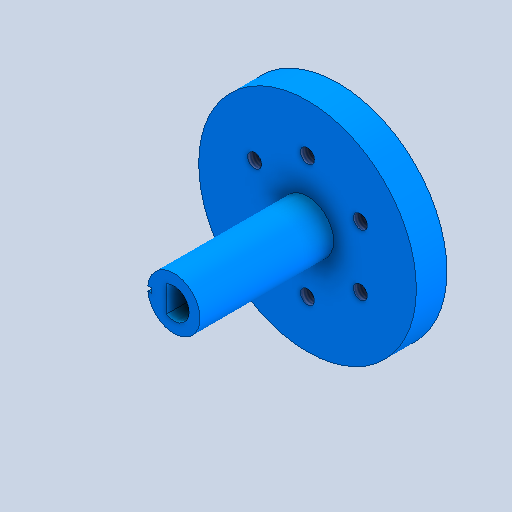
# Autodesk Inventor part: E_01
Saved by Autodesk Inventor 2024.3 (Build 283343000, 343)
## iProperties
Created: 2021-11-18
Part Number: E_01
Material: PETG
Document SubType Name: Modeling
Designer: Alcatraz
Density: 1.27 g/cm^3
Appearance: Genérico
Author: Alcatraz
Autodesk Inventor part; units mm, degrees
sketch "Boceto1" plane through (0, 0, 0) normal (0, 0, 1) x (1, 0, 0)
  circle A0 centre (0, 0) radius 28.5
  dimension "DiametroJunta" = 57
  constraints: 1 centre point, 1 coincident
  measures "DiametroJunta" diameter of A0
extrude "Extrusión1" add sketch "Boceto1" along normal blind 8
sketch "Boceto2" plane through (0, 0, 8) normal (0, 0, 1) x (1, 0, 0)
  circle A0 centre (0, 0) radius 6.8425
  dimension "DiametroEje" = 13.685
  constraints: 1 centre point, 1 coincident
  measures "DiametroEje" diameter of A0
extrude "Extrusión2" add sketch "Boceto2" along normal blind 35
sketch "Boceto3" plane through (0, 0, 43) normal (0, 0, 1) x (1, 0, 0)
  arc A0 (-2, -3.4641) -> (-2, 3.4641) centre (0, 0) ccw
  line L0 (-2, 3.4641) -> (-2, -3.4641)
  circle A1 centre (0, 0) radius 6.8425 projected
  point P0 (2, -3.4641)
  point P1 (2, 3.4641)
  dimension "DiametroEntrada" = 8
  dimension "d21" = 2
  constraints: 4 point on circle, 2 end point, 1 centre point, 1 coincident, 1 concentric, 1 vertical
  measures "DiametroEntrada" diameter of A0
  measures "d21" distance from line of point (0, 0) L0
extrude "Extrusión3" cut sketch "Boceto3" against normal blind 34.5 contours L0 A0
ref_plane "Plano de trabajo1" through (6.8425, 0, 8) normal (1, 0, 0) x (0, 1, 0)
ref_plane "Plano de trabajo2" through (-6.8425, 0, 8) normal (1, 0, 0) x (0, 1, 0)
sketch "Boceto5" plane through (-6.8425, 0, 8) normal (1, 0, 0) x (0, 1, 0)
  line L0 (6.8425, 35) -> (-6.8425, 35) projected
  line L1 (0, 35) -> (0, 10)
  circle A0 centre (0, 10) radius 1.4978
  line L2 (-0.6, 27.4718) -> (0.6, 27.4718)
  line L3 (0.6, 27.4718) -> (0.6, 35)
  line L4 (0.6, 35) -> (-0.6, 35)
  line L5 (-0.6, 35) -> (-0.6, 27.4718)
  line L6 (-0.6, 27.4718) -> (0.6, 35) construction
  line L7 (0.6, 27.4718) -> (-0.6, 35) construction
  point P0 (0, -8)
  point P1 (0, 31.2359)
  dimension "d54" = 25
  dimension "d91" = 1.2
  constraints: 14 end point, 3 midpoint, 2 parallel, 2 point on line, 1 centre point, 1 coincident, 1 horizontal, 1 perpendicular, 1 vertical
  measures "d54" distance of L1.start L1.end
  measures "d91" distance of L4.end L3.end
hole "Agujero2" at (-6.8425, 0, 18) direction (1, 0, 0) diameter 3.6881 depth 6 tip angle 118 thread size "M4.5x0.75" class "6H" standard "ISO Metric profile"
sketch "Boceto7" plane through (0, 0, 0) normal (0, 0, -1) x (-1, 0, 0)
  arc A0 (2, 3.4641) -> (2, -3.4641) centre (0, 0) ccw projected
  circle A1 centre (0, 16) radius 5
  dimension "d35" = 10
  dimension "d49" = 16
  constraints: 1 centre point
  measures "d35" diameter of A1
  measures "d49" distance of A1.centre point (0, 0)
ref_plane "Plano de trabajo3" through (0, 22.5, 15) normal (0, 0, -1) x (-1, 0, 0)
ref_plane "Plano de trabajo4" through (0, 11, 8) normal (0, 0, -1) x (-1, 0, 0)
sketch "Boceto9" plane through (0, 11, 8) normal (0, 0, -1) x (-1, 0, 0)
  circle A0 centre (0, 0) radius 2.5
  point P0 (0, -11)
  dimension "d70" = 5
  constraints: 1 centre point
  measures "d70" diameter of A0
hole "Agujero6" at (0, 16, 0) direction (0, 0, 1) diameter 3.6881 depth 13 thread size "M4.5x0.75" class "6H" standard "ISO Metric profile"
pattern_circular "Patrón circular6" count 6 over 360 about axis through (0, 0, 8) along (0, 0, 1) of "Agujero6"
extrude "Extrusión6" add sketch "Boceto5" along normal blind 1 contours L3 L2 L1 L0 | L1 L2 L5 L0
extrude "Extrusión7" cut sketch "Boceto5" along normal blind 1 contours L3 L2 L1 L0 | L1 L2 L5 L0
equation "\"d21\" = 0.25 * DiametroEntrada"
